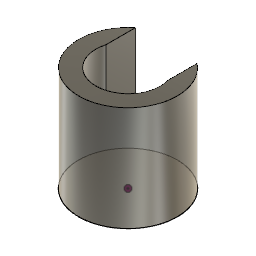
Motor Cup Wedge (Autodesk Fusion 360 design; units mm, degrees)
Autodesk Fusion 360 part; units mm, degrees
sketch "Sketch1" plane through (0, 0, 0) normal (0, 0, 1) x (1, 0, 0)
  circle A0 centre (0, 0) radius 4
  dimension "d7" = 8
  constraint coincident A0.centre origin
  measures "d7" diameter of A0
extrude "Extrude2" add sketch "Sketch1" along normal blind 8.5 makes body 1
extrude "Extrude1" add sketch "Sketch1" along normal blind 8.5 separate body makes body 2
sketch "Sketch2" plane through (0, 0, 8.5) normal (0, 0, 1) x (-1, 0, 0)
  circle A0 centre (0, 0) radius 4
  circle A1 centre (0, 0) radius 2.6
  dimension "d12" = 5.2
  constraint coincident A0.centre A1.centre
  measures "d12" diameter of A1
extrude "Extrude3" cut sketch "Sketch2" against normal blind 108.5 contours A1 bodies 1 2
sketch "Sketch3" plane through (0, 0, 0) normal (0, 1, 0) x (1, 0, 0)
  line L0 (-2.5, 0) -> (2.5, 0)
  line L1 (2.5, 0) -> (2.5, -8.5)
  line L2 (2.5, -8.5) -> (-2.5, -8.5)
  line L3 (-2.5, -8.5) -> (-2.5, 0)
  dimension "d15" = 5
  dimension "d16" = 8.5
  constraint horizontal L0
  constraint vertical L1
  constraint horizontal L2
  constraint vertical L3
  measures "d15" distance of L0.start L0.end
  measures "d16" distance of L0.start L2.end
extrude "Extrude4" cut sketch "Sketch3" along normal blind 102.6 bodies 1 2
equation "outer_radius = 4 mm"
equation "shaft_hole_radius = 2.6 mm"
equation "screw_hole_length = length"
equation "length = 8.5 mm"
equation "extra = 100 mm"
equation "screw_hole_width = 5 mm"
equation "d7 = outer_radius * 2"
equation "d8 = length"
equation "d10 = length"
equation "d12 = shaft_hole_radius * 2"
equation "d13 = -( length + extra )"
equation "d15 = screw_hole_width"
equation "d16 = screw_hole_length"
equation "d17 = shaft_hole_radius + extra"
